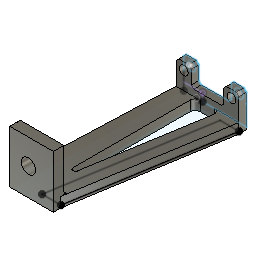
horizontal endstop holder v5 (Autodesk Fusion 360 design; units mm, degrees)
Autodesk Fusion 360 part; units mm, degrees
sketch "Sketch1" plane through (0, 0, 0) normal (0, 1, 0) x (1, 0, 0)
  line L0 (0, 0) -> (15, 0)
  line L1 (15, 0) -> (15, -20)
  line L2 (15, -20) -> (0, -20)
  line L3 (0, -20) -> (0, 0)
  line L4 (15, -10) -> (5, -10)
  circle A0 centre (5, -10) radius 2.85
  dimension "d1" = 15
  dimension "d2" = 20
  dimension "d3" = 10
  dimension "d4" = 5.7
  constraint horizontal L0
  constraint vertical L1
  constraint horizontal L2
  constraint vertical L3
  constraint coincident L0.start L3.end
  constraint midpoint L1 L4.start
  constraint perpendicular L1 L4
  constraint coincident L4.end A0.centre
  measures "d1" distance of L0.start L0.end
  measures "d2" distance of L0.start L2.end
  measures "d3" distance of L4.start L4.end
  measures "d4" diameter of A0
extrude "Extrude1" add sketch "Sketch1" along normal blind 3
sketch "Sketch2" plane through (0, 3, 0) normal (0, 1, 0) x (-1, 0, 0)
  circle A0 centre (-5, 10) radius 2.85
  line L0 (0, 20) -> (-15, 20)
  line L1 (-15, 20) -> (-15, 0)
  line L2 (-15, 0) -> (0, 0)
  line L3 (0, 0) -> (0, 20)
  line L4 (0, 0) -> (0, 3)
  line L5 (-7.5, 3) -> (-7.5, 0)
  line L6 (-7.5, 3) -> (0, 3)
  line L7 (0, 0) -> (-7.5, 0)
  constraint vertical L4
  constraint coincident L3 L4.end
  constraint perpendicular L3 L6
  constraint coincident L2.end L3.start
  constraint perpendicular L5 L7
extrude "Extrude2" add sketch "Sketch2" along normal blind 64 contours L2 L3 L4 L5 L6 L7
sketch "Sketch3" plane through (0, 67, 0) normal (0, 1, 0) x (-1, 0, 0)
  line L0 (-7.5, 0) -> (0, 0)
  line L1 (0, 0) -> (0, 3)
  line L2 (-7.5, 0) -> (-5, 0)
  circle A0 centre (-22, 10) radius 1.75
  line L3 (0, 0) -> (0, 7)
  line L4 (-24, 13) -> (-25, 12)
  line L5 (-25, 12) -> (-25, 8)
  line L6 (-20, 13) -> (-19.0202, 12.0202)
  line L7 (-20, 13) -> (-24, 13)
  line L8 (-25, 8) -> (-25, 0)
  line L9 (-25, 0) -> (-7.5, 0)
  line L10 (-2, 10) -> (-2.2292, 10)
  circle A1 centre (-3, 10) radius 1.75
  line L11 (-4, 13) -> (-5, 13)
  line L12 (-5, 13) -> (-6, 12)
  line L13 (0, 7) -> (0, 12)
  line L14 (0, 12) -> (-1, 13)
  line L15 (-4, 13) -> (-1, 13)
  line L16 (-19.0202, 12.0202) -> (-19.0202, 6.4963)
  line L17 (-19.0202, 6.4963) -> (-18.0441, 5.5202)
  line L18 (-6, 12) -> (-6, 6.5)
  line L19 (-6, 6.5) -> (-7, 5.5)
  line L20 (-7, 5.5) -> (-18.0441, 5.5202)
  line L21 (-7.5, 3) -> (-7.5, 0)
  line L22 (0, 3) -> (-7.5, 3)
  dimension "d10" = 3.5
  dimension "d13" = 3.5
  constraint coincident L0 L2.end
  constraint coincident L0.start L2.start
  constraint coincident L0.end L1.start
  constraint perpendicular L0 L3
  constraint parallel L5 L8
  constraint parallel L11 L15
  constraint vertical L16
  constraint perpendicular L4 L17
  constraint vertical L18
  measures "d10" diameter of A0
  measures "d13" diameter of A1
extrude "Extrude3" add sketch "Sketch3" against normal blind 3 contours L0 L1 L2 L3 L21 L22 | L3 L4 L5 L6 L7 L8 L9 L11 L12 L13 L14 L15 L16 L17 L18 L19 L20 L21 L22 | A0 | A1
sketch "Sketch4" plane through (0, 0, 0) normal (0, 0, -1) x (1, 0, 0)
  line L0 (7.5, -64) -> (7.5, -3)
  line L1 (7.5, -3) -> (15, -3)
  line L2 (15, -3) -> (15, 0)
  line L3 (15, 0) -> (0, 0)
  line L4 (0, 0) -> (0, -67)
  line L5 (0, -67) -> (25, -67)
  line L6 (25, -67) -> (25, -64)
  line L7 (25, -64) -> (7.5, -64)
  line L8 (15, -3) -> (25, -64)
  line L9 (25, -64) -> (17.5, -64)
  line L10 (17.5, -64) -> (7.5, -3)
  line L11 (15, -3) -> (7.5, -3)
  dimension "d15" = 7.5
  constraint coincident L1.end L2.start
  constraint coincident L6.end L7.start
  constraint perpendicular L6 L9
  constraint coincident L0.end L1.start
  measures "d15" distance of L6.end L9.end
extrude "Extrude4" add sketch "Sketch4" against normal blind 3 contours L1 L7 L8 L9 L10 L11
fillet "Fillet1" radius 1 1 edges at (7.5, 3, 1.5)
extrude "Extrude5" cut sketch "Sketch3" against normal blind 3 contours A0
extrude "Extrude6" cut sketch "Sketch3" against normal blind 3 contours A1
fillet "Fillet2" radius 2 1 edges at (7.5, 64, 1.5)
fillet "Fillet3" radius 2 1 edges at (17.5, 64, 1.5)
sketch "Sketch5" plane through (0, 0, 0) normal (0, 0, -1) x (1, 0, 0)
  line L0 (0, 0) -> (0, -67)
  line L1 (0, 0) -> (-2.5, 0)
  line L2 (-2.5, 0) -> (0, -67)
  dimension "d28" = 2.5
  constraint coincident L0.start L1.start
  constraint vertical L0
  constraint perpendicular L0 L1
  measures "d28" distance of L0.start L1.end
extrude "Extrude7" add sketch "Sketch5" against normal blind 3
sketch "Sketch6" plane through (0, 0, 3) normal (0, 0, 1) x (-1, 0, 0)
  line L0 (-9.5, -64) -> (0, -64)
  line L1 (0, -64) -> (0, -67)
  line L2 (0, -67) -> (2.5, 0)
  line L3 (2.5, 0) -> (0, 0)
  line L4 (0, 0) -> (0, -3)
  line L5 (0, -3) -> (-15, -3)
  line L6 (-15, -3) -> (-25, -64)
  line L7 (-25, -64) -> (-15.1454, -64)
  arc A0 (-17.1191, -61.6764) -> (-15.1454, -64) centre (-15.1454, -62) ccw
  line L8 (-17.1191, -61.6764) -> (-9.4868, -15.1196)
  arc A1 (-7.5, -15.2814) -> (-9.4868, -15.1196) centre (-8.5, -15.2814) ccw
  line L9 (-7.5, -15.2814) -> (-7.5, -62)
  arc A2 (-9.5, -64) -> (-7.5, -62) centre (-9.5, -62) ccw
  line L10 (0, 0) -> (0, -3)
  line L11 (0, -3) -> (2.3881, -3)
  line L12 (2.3881, -3) -> (2.5, 0)
  line L13 (0, 0) -> (2.5, 0)
  constraint coincident L3.end L4.start
  constraint coincident L4.end L5.start
  constraint coincident L2 L11.end
  constraint perpendicular L4 L11
  constraint coincident L2.end L3.start
extrude "Extrude8" add sketch "Sketch6" along normal blind 17 contours L2 L3 L4 L10 L11 L12 L13
extrude "Extrude9" add 1 faces at (1.6667, 27.4271, 0) along direction (0, 0, -1) blind 1
extrude "Extrude10" add 1 faces at (12.6061, 3, 11.1416) along direction (0, 1, 0) blind 1.2
fillet "Fillet4" radius 1 1 edges at (6.3284, 4.2, 3)
